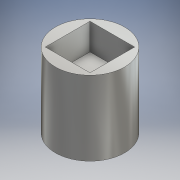
# Autodesk Inventor part: Enclosure
Saved by Autodesk Inventor 2016 (Build 200138000, 138)
## iProperties
Created: 2016-04-14
Part Number: Enclosure
Material: Generic
Document SubType Name: Modeling
Designer: Andres
Density: 1 g/cm^3
Appearance: Aluminum - Polished
Author: Andres
Autodesk Inventor part; units mm, degrees
ref_plane "YZ Plane" through (0, 0, 0) normal (1, 0, 0) x (0, 1, 0)
ref_plane "XZ Plane" through (0, 0, 0) normal (0, 1, 0) x (-1, 0, 0)
ref_plane "XY Plane" through (0, 0, 0) normal (0, 0, 1) x (1, 0, 0)
sketch "Sketch1" plane through (0, 0, 0) normal (0, 0, 1) x (1, 0, 0)
  circle A0 centre (0, 0) radius 32.5
  dimension "d32" = 65
  constraints: 1 centre point
  measures "d32" diameter of A0
extrude "Extrusion1" add sketch "Sketch1" along normal blind 70
sketch "Sketch2" plane through (0, 0, 70) normal (0, 0, 1) x (1, 0, 0)
  line L0 (-21, 21) -> (21, 21)
  line L1 (21, 21) -> (21, -21)
  line L2 (21, -21) -> (-21, -21)
  line L3 (-21, -21) -> (-21, 21)
  point P0 (0, 0)
  point P1 (-21, 0)
  point P2 (0, 21)
  dimension "d4" = 42
  dimension "d5" = 42
  constraints: 8 end point, 2 midpoint, 2 parallel, 1 horizontal, 1 horizontal alignment, 1 perpendicular, 1 vertical alignment
  measures "d4" distance of L0.end L1.end
  measures "d5" distance of L0.start L0.end
extrude "Extrusion2" cut sketch "Sketch2" against normal blind 25
sketch "Sketch3" plane through (0, 0, 45) normal (0, 0, 1) x (1, 0, 0)
  point P0 (0, 0)
sketch "Sketch4" plane through (0, 0, 0) normal (0, 0, -1) x (-1, 0, 0)
  circle A0 centre (0, 0) radius 5
  dimension "d8" = 10
  constraints: 1 centre point, 1 coincident
  measures "d8" diameter of A0
extrude "Extrusion3" cut sketch "Sketch4" against normal blind 10
sketch "Sketch5" plane through (0, 0, 10) normal (0, 0, -1) x (-1, 0, 0)
  circle A0 centre (0, 0) radius 2.5
  dimension "d11" = 5
  constraints: 1 centre point, 1 coincident
  measures "d11" diameter of A0
extrude "Extrusion4" cut sketch "Sketch5" against normal blind 35
sketch "Sketch6" plane through (0, 0, 0) normal (0, 0, -1) x (-1, 0, 0)
  line L0 (-7.5, -7.5) -> (7.5, -7.5)
  line L1 (7.5, -7.5) -> (7.5, 7.5)
  line L2 (7.5, 7.5) -> (-7.5, 7.5)
  line L3 (-7.5, 7.5) -> (-7.5, -7.5)
  point P0 (0, 0)
  point P1 (-7.5, 0)
  point P2 (0, 7.5)
  dimension "d14" = 15
  dimension "d15" = 15
  constraints: 8 end point, 2 midpoint, 2 parallel, 1 horizontal, 1 horizontal alignment, 1 perpendicular, 1 vertical alignment
  measures "d14" distance of L0.end L1.end
  measures "d15" distance of L0.start L0.end
extrude "Extrusion5" cut sketch "Sketch6" against normal blind 2.5
ref_plane "Work Plane2" through (0, 0, 10) normal (0, 0, -1) x (-1, 0, 0)
sketch "Sketch9" plane through (0, 0, 0) normal (0, 0, -1) x (-1, 0, 0)
  point P0 (0, 0)
ref_plane "Work Plane3" through (-21, 32.5, 70) normal (0, -1, 0) x (1, 0, 0)
ref_plane "Work Plane4" through (-21, -32.5, 70) normal (0, 1, 0) x (1, 0, 0)
ref_plane "Work Plane5" through (32.5, -21, 70) normal (-1, 0, 0) x (0, 0, 1)
ref_plane "Work Plane6" through (-32.5, -21, 70) normal (1, 0, 0) x (0, 0, -1)
ref_plane "Work Plane7" through (20, -7.5, 0) normal (-1, 0, 0) x (0, 0, 1)
sketch "Sketch15" plane through (20, -7.5, 0) normal (-1, 0, 0) x (0, 0, 1)
  line L0 (0, 40) -> (0, -25) projected
  line L1 (24.8794, -5) -> (-0.0206, -5)
  line L2 (-0.0206, -5) -> (-0.0206, 20)
  line L3 (-0.0206, 20) -> (24.8794, 20)
  line L4 (24.8794, 20) -> (24.8794, -5)
  point P0 (0, 7.5)
  dimension "d63" = 24.9
  dimension "d64" = 12.5
  dimension "d65" = 12.5
  constraints: 8 end point, 2 parallel, 1 horizontal, 1 perpendicular
  measures "d63" distance of L2.end L3.end
  measures "d64" distance from line of L3 point (0, 7.5)
  measures "d65" distance from line of point (0, 7.5) L1
extrude "Extrusion10" cut sketch "Sketch15" against normal blind 5
ref_plane "Work Plane8" through (-7.5, 20, 0) normal (0, -1, 0) x (1, 0, 0)
sketch "Sketch16" plane through (-7.5, 20, 0) normal (0, -1, 0) x (1, 0, 0)
  line L0 (-5, 0) -> (20, 0)
  line L1 (20, 0) -> (20, 24.9)
  line L2 (20, 24.9) -> (-5, 24.9)
  line L3 (-5, 24.9) -> (-5, 0)
  point P0 (7.5, 0)
  dimension "d69" = 12.5
  dimension "d70" = 12.5
  dimension "d71" = 24.9
  constraints: 8 end point, 2 parallel, 1 horizontal, 1 perpendicular
  measures "d69" distance from line of L3 point (7.5, 0)
  measures "d70" distance from line of L1 point (7.5, 0)
  measures "d71" distance of L2.end L0.start
extrude "Extrusion11" cut sketch "Sketch16" against normal blind 5
ref_plane "Work Plane9" through (-20, -7.5, 0) normal (1, 0, 0) x (0, 0, -1)
sketch "Sketch17" plane through (-20, -7.5, 0) normal (1, 0, 0) x (0, 0, -1)
  line L0 (0.1016, 20) -> (-24.7984, 20)
  line L1 (-24.7984, 20) -> (-24.7984, -5)
  line L2 (-24.7984, -5) -> (0.1016, -5)
  line L3 (0.1016, -5) -> (0.1016, 20)
  point P0 (0, 7.5)
  dimension "d75" = 12.5
  dimension "d76" = 12.5
  dimension "d77" = 24.9
  constraints: 8 end point, 2 parallel, 1 horizontal, 1 perpendicular
  measures "d75" distance from line of L0 point (0, 7.5)
  measures "d76" distance from line of L2 point (0, 7.5)
  measures "d77" distance of L0.start L0.end
extrude "Extrusion12" cut sketch "Sketch17" against normal blind 5
ref_plane "Work Plane10" through (-7.5, -20, 0) normal (0, 1, 0) x (1, 0, 0)
sketch "Sketch18" plane through (-7.5, -20, 0) normal (0, 1, 0) x (1, 0, 0)
  line L0 (20, 0) -> (-5, 0) projected
  line L1 (-5, 0) -> (20, 0)
  line L2 (20, 0) -> (20, -24.9)
  line L3 (20, -24.9) -> (-5, -24.9)
  line L4 (-5, -24.9) -> (-5, 0)
  point P0 (7.5, 0)
  dimension "d81" = 24.9
  dimension "d82" = 12.5
  dimension "d83" = 12.5
  constraints: 8 end point, 2 parallel, 1 horizontal, 1 perpendicular, 1 point on line
  measures "d81" distance of L3.end L1.start
  measures "d82" distance from line of L4 point (7.5, 0)
  measures "d83" distance from line of L2 point (7.5, 0)
extrude "Extrusion13" cut sketch "Sketch18" against normal blind 5
body "Solid1"
